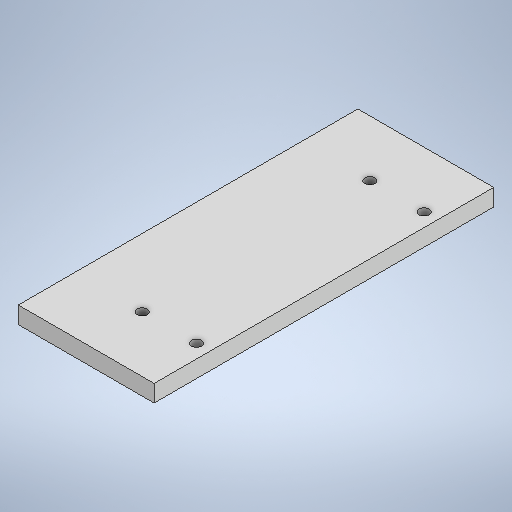
# Autodesk Inventor part: Base
Saved by Autodesk Inventor 2025.2 (Build 292293000, 293)
## iProperties
Created: 2025-01-27
Part Number: Base
Material: Genérico
Document SubType Name: Modeling
Designer: alex
Density: 1 g/cm^3
Appearance: Valor por defecto
Author: alex
Autodesk Inventor part; units mm, degrees
ref_plane "YZ Plane" through (0, 0, 0) normal (1, 0, 0) x (0, 1, 0)
ref_plane "XZ Plane" through (0, 0, 0) normal (0, 1, 0) x (-1, 0, 0)
ref_plane "XY Plane" through (0, 0, 0) normal (0, 0, 1) x (1, 0, 0)
sketch "Boceto1" plane through (0, 0, 0) normal (0, 1, 0) x (-1, 0, 0)
  line L0 (0, 0) -> (40, 0)
  line L1 (40, 0) -> (40, -100)
  line L2 (40, -100) -> (0, -100)
  line L3 (0, -100) -> (0, 0)
  circle A0 centre (19.95, -16.5) radius 1.5
  circle A1 centre (4, -16.5) radius 1.5
  circle A2 centre (19.95, -83.5) radius 1.5
  circle A3 centre (4, -83.5) radius 1.5
  point P0 (20, 0)
  dimension "d0" = 40
  dimension "d1" = 100
  dimension "d2" = 3
  dimension "d3" = 3
  dimension "d4" = 3
  dimension "d5" = 3
  dimension "d6" = 16.5
  dimension "d7" = 4
  dimension "d8" = 15.95
  dimension "d9" = 16.5
  dimension "d10" = 16.5
  dimension "d11" = 16.5
  dimension "d12" = 4
  dimension "d13" = 15.95
  constraints: 8 end point, 4 centre point, 2 parallel, 1 horizontal, 1 midpoint, 1 perpendicular
  measures "d0" distance of L1.end L2.end
  measures "d1" distance of L0.end L1.end
  measures "d2" diameter of A0
  measures "d3" diameter of A1
  measures "d4" diameter of A2
  measures "d5" diameter of A3
  measures "d6" distance from line of L0 A1.centre
  measures "d7" distance from line of L3 A1.centre
  measures "d8" distance of A0.centre A1.centre
  measures "d9" vertical distance of point (20, 0) A0.centre
  measures "d10" distance from line of L2 A2.centre
  measures "d11" distance from line of L2 A3.centre
  measures "d12" distance from line of L3 A3.centre
  measures "d13" distance of A3.centre A2.centre
extrude "Extrusión1" add sketch "Boceto1" along normal blind 5
